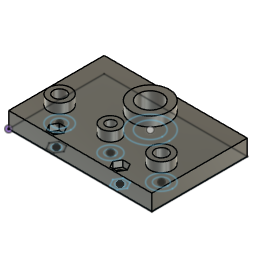
Minifix Template p1 (Autodesk Fusion 360 design; units mm, degrees)
Autodesk Fusion 360 part; units mm, degrees
sketch "Sketch1" plane through (0, 0, 0) normal (0, 0, 1) x (1, 0, 0)
  line L0 (0, 0) -> (90, 0)
  line L1 (90, 0) -> (90, 60)
  line L2 (90, 60) -> (0, 60)
  line L3 (0, 60) -> (0, 0)
  circle A0 centre (45, 19) radius 3
  circle A1 centre (13, 19) radius 4
  circle A2 centre (77, 19) radius 4
  circle A3 centre (45, 44) radius 7.5
  line L4 (22.6906, 1) -> (27.3094, 1)
  line L5 (27.3094, 1) -> (29.6188, 5)
  line L6 (29.6188, 5) -> (27.3094, 9)
  line L7 (27.3094, 9) -> (22.6906, 9)
  line L8 (22.6906, 9) -> (20.3812, 5)
  line L9 (20.3812, 5) -> (22.6906, 1)
  line L10 (67.3524, 8.9748) -> (62.7339, 9.0247)
  line L11 (62.7339, 9.0247) -> (60.3815, 5.0499)
  line L12 (60.3815, 5.0499) -> (62.6476, 1.0252)
  line L13 (62.6476, 1.0252) -> (67.2661, 0.9753)
  line L14 (67.2661, 0.9753) -> (69.6185, 4.9501)
  line L15 (69.6185, 4.9501) -> (67.3524, 8.9748)
  circle A4 centre (25, 5) radius 2.5
  circle A5 centre (65, 5) radius 2.5
  circle A6 centre (45, 44) radius 12
  circle A7 centre (77, 19) radius 7
  circle A8 centre (45, 19) radius 6
  circle A9 centre (13, 19) radius 7
  point P0 (25, 5)
  point P1 (65, 5)
  dimension "d4" = 90
  dimension "d5" = 60
  dimension "d6" = 45
  dimension "d7" = 32
  dimension "d8" = 32
  dimension "d9" = 19
  dimension "d10" = 19
  dimension "d11" = 19
  dimension "d12" = 25
  dimension "d16" = 8
  dimension "d17" = 25
  dimension "d19" = 5
  dimension "d20" = 8
  dimension "d21" = 40
  dimension "d22" = 5
  constraint horizontal L0
  constraint vertical L1
  constraint horizontal L2
  constraint vertical L3
  constraint coincident L0.start L3.end
  constraint parallel L0 L4
  constraint coincident P0 A4.centre
  constraint coincident P1 A5.centre
  constraint concentric A3 A6
  constraint concentric A2 A7
  constraint concentric A0 A8
  constraint concentric A1 A9
  measures "d4" distance of L1.end L2.end
  measures "d5" distance of L0.end L1.end
  measures "d6" distance of L3 A0.centre
  measures "d7" horizontal distance of A0.centre A1.centre
  measures "d8" horizontal distance of A0.centre A2.centre
  measures "d9" distance of L0 A1.centre
  measures "d10" distance of L0 A0.centre
  measures "d11" distance of L0 A2.centre
  measures "d12" distance of A0.centre A3.centre
  measures "d16" distance of L4 L7
  measures "d17" distance of L3 P0
  measures "d19" distance of L0 P0
  measures "d20" distance of L10 L13
  measures "d21" distance of P0 P1
  measures "d22" distance of L0 P1
extrude "Extrude1" add sketch "Sketch1" along normal blind 10 contours L0 L1 L2 L3 | L4 L5 L6 L7 L8 L9 | L10 L11 L12 L13 L14 L15 | A6 | A7 | A8 | A9
extrude "Extrude2" cut sketch "Sketch1" along normal blind 10 and the other way blind -6 contours L4 L5 L6 L7 L8 L9 | L10 L11 L12 L13 L14 L15
extrude "Extrude3" add sketch "Sketch1" along normal blind 16 contours A6 | A7 | A8 | A9
